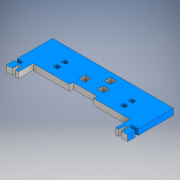
# Autodesk Inventor part: MonsterHolderBase
Saved by Autodesk Inventor 2019 (Build 230136000, 136)
## iProperties
Created: 2018-12-04
Part Number: MonsterHolderBase
Material: Generic
Document SubType Name: Modeling
Designer: Administrator
Density: 1 g/cm^3
Appearance: Default
Author: Administrator
Autodesk Inventor part; units mm, degrees
ref_plane "YZ Plane" through (0, 0, 0) normal (1, 0, 0) x (0, 1, 0)
ref_plane "XZ Plane" through (0, 0, 0) normal (0, 1, 0) x (-1, 0, 0)
ref_plane "XY Plane" through (0, 0, 0) normal (0, 0, 1) x (1, 0, 0)
sketch "Sketch1" plane through (0, 0, 0) normal (0, 1, 0) x (-1, 0, 0)
  line L0 (0, 0) -> (41.91, 0)
  line L1 (41.91, 0) -> (41.91, -127)
  line L2 (41.91, -127) -> (0, -127)
  line L3 (0, -127) -> (0, 0)
  dimension "d0" = 127
  dimension "d1" = 41.91
  constraints: 8 end point, 2 parallel, 1 horizontal, 1 perpendicular
  measures "d0" distance of L0.end L1.end
  measures "d1" distance of L1.end L2.end
extrude "Extrusion1" add sketch "Sketch1" along normal blind 6.35
sketch "Sketch2" plane through (0, 6.35, 0) normal (0, 1, 0) x (1, 0, 0)
  line L0 (-25.4, 26.035) -> (-21.59, 26.035)
  line L1 (-21.59, 26.035) -> (-21.59, 30.48)
  line L2 (-21.59, 30.48) -> (-25.4, 30.48)
  line L3 (-25.4, 30.48) -> (-25.4, 26.035)
  line L4 (-25.4, 96.52) -> (-21.59, 96.52)
  line L5 (-21.59, 96.52) -> (-21.59, 100.965)
  line L6 (-21.59, 100.965) -> (-25.4, 100.965)
  line L7 (-25.4, 100.965) -> (-25.4, 96.52)
  line L8 (0, 0) -> (0, 127) projected
  line L9 (-41.91, 0) -> (0, 0) projected
  line L10 (0, 127) -> (-41.91, 127) projected
  line L11 (-17.018, 26.035) -> (-13.208, 26.035)
  line L12 (-13.208, 26.035) -> (-13.208, 30.48)
  line L13 (-13.208, 30.48) -> (-17.018, 30.48)
  line L14 (-17.018, 30.48) -> (-17.018, 26.035)
  line L15 (-17.018, 96.52) -> (-13.208, 96.52)
  line L16 (-13.208, 96.52) -> (-13.208, 100.965)
  line L17 (-13.208, 100.965) -> (-17.018, 100.965)
  line L18 (-17.018, 100.965) -> (-17.018, 96.52)
  line L19 (-41.91, 127) -> (-41.91, 0) projected
  dimension "d5" = 4.445
  dimension "d6" = 3.81
  dimension "d7" = 4.445
  dimension "d8" = 26.035
  dimension "d9" = 26.035
  dimension "d12" = 4.445
  dimension "d13" = 4.445
  dimension "d14" = 3.81
  dimension "d15" = 26.035
  dimension "d16" = 26.035
  dimension "d18" = 8.382
  dimension "d36" = 16.51
  constraints: 32 end point, 8 parallel, 4 horizontal, 4 perpendicular, 4 point on line
  measures "d5" distance of L0.end L1.end
  measures "d6" distance of L0.start L0.end
  measures "d7" distance of L4.end L5.end
  measures "d8" distance between parallel lines of L9 L0
  measures "d9" distance between parallel lines of L10 L6
  measures "d12" distance of L15.end L16.end
  measures "d13" distance of L11.end L12.end
  measures "d14" distance of L12.end L13.end
  measures "d15" distance between parallel lines of L9 L11
  measures "d16" distance between parallel lines of L10 L17
  measures "d18" distance between parallel lines of L7 L18
  measures "d36" distance between parallel lines of L19 L7
extrude "Extrusion3" cut sketch "Sketch2" against normal blind 6.35 contours L3 L2 L1 L0 | L7 L6 L5 L4 | L14 L13 L12 L11 | L18 L17 L16 L15
sketch "Sketch4" plane through (0, 6.35, 0) normal (0, 1, 0) x (1, 0, 0)
  line L0 (-41.91, 127) -> (-41.91, 0) projected
  line L1 (-41.91, 114.3) -> (-29.21, 114.3)
  line L2 (-29.21, 114.3) -> (-29.21, 12.7)
  line L3 (-29.21, 12.7) -> (-41.91, 12.7)
  line L4 (-41.91, 12.7) -> (-41.91, 114.3)
  line L5 (-41.91, 0) -> (0, 0) projected
  line L6 (0, 127) -> (-41.91, 127) projected
  dimension "d61" = 12.7
  dimension "d62" = 12.7
  dimension "d63" = 12.7
  constraints: 8 end point, 2 parallel, 1 horizontal, 1 perpendicular, 1 point on line
  measures "d61" distance between parallel lines of L5 L3
  measures "d62" distance between parallel lines of L6 L1
  measures "d63" distance of L2.end L3.end
sketch "Sketch6" plane through (0, 6.35, 0) normal (0, 1, 0) x (1, 0, 0)
  line L0 (0, 127) -> (-41.91, 127) projected
  line L1 (-40.3225, 127) -> (-37.1475, 127)
  line L2 (-37.1475, 127) -> (-37.1475, 120.65)
  line L3 (-37.1475, 120.65) -> (-40.3225, 120.65)
  line L4 (-40.3225, 120.65) -> (-40.3225, 127)
  line L5 (-41.91, 0) -> (0, 0) projected
  line L6 (-40.3225, 0) -> (-37.1475, 0)
  line L7 (-37.1475, 0) -> (-37.1475, 6.35)
  line L8 (-37.1475, 6.35) -> (-40.3225, 6.35)
  line L9 (-40.3225, 6.35) -> (-40.3225, 0)
  line L10 (-41.91, 127) -> (-41.91, 0) projected
  point P0 (-41.91, 107.95)
  dimension "d37" = 1.5875
  dimension "d38" = 6.35
  dimension "d39" = 3.175
  dimension "d40" = 6.35
  constraints: 16 end point, 4 parallel, 4 point on line, 2 horizontal, 2 perpendicular
  measures "d37" distance between parallel lines of L10 L4
  measures "d38" distance of L3.end L1.start
  measures "d39" distance between parallel lines of L4 L2
  measures "d40" distance from line of L8 L6.end
extrude "Extrusion6" cut sketch "Sketch6" against normal blind 25.4
ref_plane "Work Plane1" through (-41.91, 0, -101.6) normal (-1, 0, 0) x (0, 0, 1)
sketch "Sketch7" plane through (-41.91, 0, -101.6) normal (-1, 0, 0) x (0, 0, 1)
  line L0 (88.9, 6.35) -> (88.9, 0) projected
  line L1 (101.6, 0) -> (101.6, 6.35) projected
  line L2 (88.9, 6.35) -> (101.6, 6.35)
  line L3 (101.6, 6.35) -> (101.6, 0)
  line L4 (101.6, 0) -> (88.9, 0)
  line L5 (88.9, 0) -> (88.9, 6.35)
  line L6 (101.6, 0) -> (-25.4, 0) projected
  line L7 (-25.4, 6.35) -> (-12.7, 6.35)
  line L8 (-12.7, 6.35) -> (-12.7, 0)
  line L9 (-12.7, 0) -> (-25.4, 0)
  line L10 (-25.4, 0) -> (-25.4, 6.35)
  point P0 (-6.35, 0)
  point P1 (-19.05, 6.35)
  dimension "d66" = 12.7
  constraints: 16 end point, 4 parallel, 2 horizontal, 2 perpendicular, 1 point on line
  measures "d66" distance between parallel lines of L10 L8
extrude "Extrusion10" add sketch "Sketch7" along normal blind 6.35
ref_plane "Work Plane2" through (-48.26, 0, -101.6) normal (-1, 0, 0) x (0, 0, 1)
extrude "Extrusion9" cut sketch "Sketch4" against normal blind 6.35
sketch "Sketch10" plane through (-48.26, 0, -101.6) normal (-1, 0, 0) x (0, 0, 1)
  line L0 (95.25, 0) -> (92.075, 0)
  line L1 (92.075, 0) -> (92.075, 6.35)
  line L2 (92.075, 6.35) -> (95.25, 6.35)
  line L3 (95.25, 6.35) -> (95.25, 0)
  line L4 (-19.05, 0) -> (-15.875, 0)
  line L5 (-15.875, 0) -> (-15.875, 6.35)
  line L6 (-15.875, 6.35) -> (-19.05, 6.35)
  line L7 (-19.05, 6.35) -> (-19.05, 0)
  line L8 (-25.4, 6.35) -> (-25.4, 0) projected
  line L9 (101.6, 0) -> (101.6, 6.35) projected
  point P0 (-12.7, 0)
  dimension "d70" = 3.175
  dimension "d72" = 3.175
  dimension "d73" = 6.35
  dimension "d74" = 6.35
  dimension "d75" = 6.35
  dimension "d76" = 6.35
  constraints: 16 end point, 4 parallel, 2 horizontal, 2 perpendicular
  measures "d70" distance between parallel lines of L3 L1
  measures "d72" distance between parallel lines of L5 L7
  measures "d73" distance between parallel lines of L8 L7
  measures "d74" distance between parallel lines of L6 L4
  measures "d75" distance between parallel lines of L9 L3
  measures "d76" distance of L2.end L0.start
extrude "Extrusion12" cut sketch "Sketch10" against normal blind 6.35
sketch "Sketch11" plane through (0, 6.35, 0) normal (0, 1, 0) x (1, 0, 0)
  line L0 (-11.43, 60.96) -> (-5.08, 60.96)
  line L1 (-5.08, 60.96) -> (-5.08, 54.61)
  line L2 (-5.08, 54.61) -> (-11.43, 54.61)
  line L3 (-11.43, 54.61) -> (-11.43, 60.96)
  line L4 (-37.1475, 0) -> (0, 0) projected
  line L5 (0, 0) -> (0, 127) projected
  line L6 (-29.21, 114.3) -> (-29.21, 12.7) projected
  dimension "d82" = 54.61
  dimension "d83" = 6.35
  dimension "d84" = 6.35
  dimension "d86" = 17.78
  constraints: 8 end point, 2 parallel, 1 horizontal, 1 perpendicular
  measures "d82" distance between parallel lines of L4 L2
  measures "d83" distance between parallel lines of L0 L2
  measures "d84" distance of L1.end L2.end
  measures "d86" distance between parallel lines of L6 L3
extrude "Extrusion13" cut sketch "Sketch11" against normal blind 6.35
sketch "Sketch12" plane through (0, 6.35, 0) normal (0, 1, 0) x (1, 0, 0)
  line L0 (-22.86, 50.673) -> (-16.51, 50.673)
  line L1 (-16.51, 50.673) -> (-16.51, 57.023)
  line L2 (-16.51, 57.023) -> (-22.86, 57.023)
  line L3 (-22.86, 57.023) -> (-22.86, 50.673)
  line L4 (-22.86, 69.977) -> (-16.51, 69.977)
  line L5 (-16.51, 69.977) -> (-16.51, 76.327)
  line L6 (-16.51, 76.327) -> (-22.86, 76.327)
  line L7 (-22.86, 76.327) -> (-22.86, 69.977)
  line L8 (-29.21, 114.3) -> (-29.21, 12.7) projected
  line L9 (-37.1475, 0) -> (0, 0) projected
  line L10 (0, 127) -> (-37.1475, 127) projected
  dimension "d90" = 6.35
  dimension "d91" = 6.35
  dimension "d92" = 6.35
  dimension "d93" = 50.673
  dimension "d94" = 6.35
  dimension "d95" = 50.673
  constraints: 16 end point, 4 parallel, 2 horizontal, 2 perpendicular, 2 point on line
  measures "d90" distance between parallel lines of L8 L3
  measures "d91" distance of L0.start L0.end
  measures "d92" distance of L0.end L1.end
  measures "d93" distance between parallel lines of L9 L0
  measures "d94" distance of L4.end L5.end
  measures "d95" distance between parallel lines of L10 L6
extrude "Extrusion14" cut sketch "Sketch12" against normal blind 6.35
sketch "Sketch13" plane through (-29.21, 6.35, -114.3) normal (-1, 0, 0) x (0, 0, 1)
  line L0 (101.6, -6.35) -> (63.5, -6.35)
  line L1 (63.5, -6.35) -> (63.5, 0)
  line L2 (63.5, 0) -> (101.6, 0)
  line L3 (101.6, 0) -> (101.6, -6.35)
  line L4 (101.6, -6.35) -> (0, -6.35) projected
  line L5 (0, 0) -> (101.6, 0) projected
  line L6 (0, -6.35) -> (38.1, -6.35)
  line L7 (38.1, -6.35) -> (38.1, 0)
  line L8 (38.1, 0) -> (0, 0)
  line L9 (0, 0) -> (0, -6.35)
  point P0 (114.3, -6.35)
  dimension "d98" = 38.1
  dimension "d99" = 38.1
  constraints: 16 end point, 4 parallel, 2 horizontal, 2 perpendicular, 1 point on line
  measures "d98" distance between parallel lines of L9 L7
  measures "d99" distance between parallel lines of L3 L1
extrude "Extrusion15" add sketch "Sketch13" along normal blind 3.81 contours L0 L1 L2 L3 | L4 L9 L5 L7
body "Solid1"
